Autodesk Fusion 360 part; units mm, degrees
(part 6 of 6)
  line L3972 (32.949444, 239.306805) -> (33.090556, 239.906528)
  line L3973 (28.328056, 253.559028) -> (28.398611, 253.594305)
  line L3974 (29.845, 285.802917) -> (29.809722, 285.697083)
  line L3975 (13.229167, 258.180417) -> (13.193889, 258.497917)
  line L3976 (27.269722, 228.75875) -> (27.199167, 228.864583)
  line L3977 (21.801667, 225.407361) -> (21.872222, 225.477917)
  line L3978 (35.665833, 285.555972) -> (35.736389, 285.59125)
  line L3979 (35.736389, 285.59125) -> (35.771667, 285.661805)
  line L3980 (35.771667, 285.661805) -> (35.806944, 285.873472)
  line L3981 (42.051111, 264.424583) -> (42.156944, 264.283472)
  line L3982 (42.156944, 264.283472) -> (42.2275, 264.248194)
  line L3983 (42.2275, 264.248194) -> (42.298056, 264.248194)
  line L3984 (41.557222, 264.847917) -> (41.733611, 264.812639)
  line L3985 (38.911389, 241.635139) -> (39.017222, 241.599861)
  line L3986 (38.382222, 243.434305) -> (38.311667, 243.68125)
  line L3987 (27.234444, 231.93375) -> (27.340278, 232.004305)
  line L3988 (25.011944, 247.244305) -> (25.611667, 247.385417)
  line L3989 (31.4325, 231.93375) -> (31.467778, 231.863194)
  line L3990 (22.154444, 225.548472) -> (22.754167, 225.548472)
  line L3991 (29.598056, 293.564028) -> (29.598056, 293.422917)
  line L3992 (30.021389, 253.559028) -> (30.056667, 253.594305)
  line L3993 (41.874722, 273.490972) -> (41.345556, 275.325417)
  line L3994 (41.345556, 275.325417) -> (40.781111, 273.490972)
  line L3995 (40.781111, 273.490972) -> (41.874722, 273.490972)
  line L3996 (28.575, 253.559028) -> (28.610278, 253.52375)
  line L3997 (29.809722, 294.763472) -> (27.798889, 294.763472)
  line L3998 (10.830278, 224.63125) -> (10.724444, 224.772361)
  line L3999 (29.421667, 293.21125) -> (29.351111, 293.175972)
  line L4000 (40.287222, 244.034028) -> (40.251944, 243.963472)
  line L4001 (34.6075, 286.367361) -> (34.466389, 286.085139)
  line L4002 (34.466389, 286.085139) -> (34.29, 285.90875)
  line L4003 (27.163889, 289.683472) -> (27.199167, 289.577639)
  line L4004 (31.608889, 225.372083) -> (31.573611, 225.336805)
  line L4005 (24.800278, 289.71875) -> (24.765, 289.648194)
  line L4006 (29.845, 232.004305) -> (31.220833, 232.004305)
  line L4007 (31.220833, 232.004305) -> (31.361944, 231.969028)
  line L4008 (26.246667, 234.826528) -> (25.611667, 234.932361)
  line L4009 (8.643056, 223.149583) -> (8.396111, 223.114305)
  line L4010 (8.396111, 223.114305) -> (6.173611, 223.114305)
  line L4011 (31.467778, 228.899861) -> (31.467778, 228.829305)
  line L4012 (23.530278, 229.852361) -> (23.565556, 229.640694)
  line L4013 (23.212778, 230.169861) -> (23.353889, 230.134583)
  line L4014 (40.3225, 233.239028) -> (40.357778, 233.168472)
  line L4015 (24.024167, 218.034306) -> (25.435278, 218.034306)
  line L4016 (17.674167, 218.034306) -> (19.085278, 218.034306)
  line L4017 (23.600833, 222.549861) -> (19.085278, 218.034306)
  line L4018 (19.085278, 218.034306) -> (24.024167, 218.034306)
  line L4019 (24.024167, 218.034306) -> (28.504444, 222.549861)
  line L4020 (29.351111, 293.175972) -> (29.421667, 293.21125)
  line L4021 (32.208611, 295.292639) -> (32.0675, 295.186805)
  line L4022 (31.785278, 287.249305) -> (31.891111, 286.790694)
  line L4023 (31.891111, 286.790694) -> (32.032222, 286.473194)
  line L4024 (32.032222, 286.473194) -> (32.243889, 286.190972)
  line L4025 (32.596667, 289.542361) -> (32.208611, 289.119028)
  line L4026 (40.181389, 253.20625) -> (40.251944, 253.20625)
  line L4027 (38.311667, 244.245694) -> (38.4175, 244.527917)
  line L4028 (31.220833, 228.723472) -> (29.845, 228.723472)
  line L4029 (23.777222, 289.648194) -> (23.741944, 289.71875)
  line L4030 (41.521944, 263.04875) -> (41.627778, 263.013472)
  line L4031 (30.1625, 294.939861) -> (30.091944, 294.834028)
  line L4032 (27.375556, 250.419305) -> (27.410833, 250.384028)
  line L4033 (27.410833, 250.384028) -> (27.446111, 250.34875)
  line L4034 (28.786667, 234.297361) -> (29.421667, 234.509028)
  line L4035 (29.421667, 234.509028) -> (30.021389, 234.79125)
  line L4036 (38.770278, 243.751805) -> (38.840833, 243.575417)
  line L4037 (35.277778, 273.490972) -> (34.148889, 273.490972)
  line L4038 (37.006389, 261.390694) -> (37.041667, 261.284861)
  line L4039 (29.845, 289.295417) -> (29.845, 285.873472)
  line L4040 (38.205833, 253.170972) -> (38.276389, 253.20625)
  line L4041 (28.151667, 227.17125) -> (28.186944, 227.277083)
  line L4042 (38.488056, 243.257917) -> (38.629167, 243.116805)
  line L4043 (39.087778, 244.915972) -> (38.735, 244.810139)
  line L4044 (38.735, 244.810139) -> (38.4175, 244.527917)
  line L4045 (38.4175, 244.527917) -> (38.311667, 244.245694)
  line L4046 (15.451667, 225.301528) -> (15.522222, 225.336805)
  line L4047 (32.138056, 237.613472) -> (31.75, 237.119583)
  line L4048 (15.522222, 225.336805) -> (15.5575, 225.372083)
  line L4049 (15.5575, 225.372083) -> (15.5575, 225.513194)
  line L4050 (35.771667, 285.661805) -> (35.736389, 285.59125)
  line L4051 (28.151667, 224.807639) -> (28.151667, 227.030139)
  line L4052 (38.205833, 294.834028) -> (38.276389, 294.869305)
  line L4053 (38.276389, 294.869305) -> (38.311667, 294.904583)
  line L4054 (38.311667, 294.904583) -> (38.311667, 295.045694)
  line L4055 (32.279167, 287.390417) -> (32.349722, 287.108194)
  line L4056 (32.349722, 287.108194) -> (32.490833, 286.755417)
  line L4057 (32.138056, 257.898194) -> (31.996944, 257.615972)
  line L4058 (29.633333, 231.93375) -> (29.739167, 232.004305)
  line L4059 (39.6875, 241.705694) -> (39.828611, 241.917361)
  line L4060 (30.656389, 280.722917) -> (30.973889, 280.687639)
  line L4061 (32.032222, 291.235694) -> (32.0675, 291.165139)
  line L4062 (32.0675, 291.165139) -> (32.138056, 291.094583)
  line L4063 (32.138056, 291.094583) -> (32.279167, 291.059305)
  line L4064 (12.170833, 227.312361) -> (12.241389, 227.347639)
  line L4065 (15.5575, 225.513194) -> (15.5575, 225.58375)
  line L4066 (15.5575, 225.58375) -> (15.522222, 225.689583)
  line L4067 (36.477222, 227.030139) -> (36.477222, 227.135972)
  line L4068 (31.079722, 295.292639) -> (30.938611, 295.257361)
  line L4069 (28.222222, 289.754028) -> (28.469167, 289.824583)
  line L4070 (35.489444, 285.59125) -> (35.595278, 285.555972)
  line L4071 (35.348333, 289.507083) -> (35.348333, 285.873472)
  line L4072 (35.348333, 289.648194) -> (35.348333, 289.577639)
  line L4073 (13.899444, 257.157361) -> (13.6525, 257.369028)
  line L4074 (29.245278, 293.705139) -> (27.798889, 293.705139)
  line L4075 (28.151667, 227.030139) -> (28.151667, 227.17125)
  line L4076 (27.093333, 289.365972) -> (27.163889, 289.471805)
  line L4077 (27.163889, 289.471805) -> (27.199167, 289.577639)
  line L4078 (38.911389, 244.386805) -> (38.770278, 244.210417)
  line L4079 (31.855833, 222.549861) -> (34.325278, 222.549861)
  line L4080 (34.325278, 222.549861) -> (34.854444, 222.549861)
  line L4081 (36.300833, 222.549861) -> (37.923611, 222.549861)
  line L4082 (28.539722, 253.594305) -> (28.469167, 253.594305)
  line L4083 (29.280556, 252.112639) -> (28.645556, 253.488472)
  line L4084 (31.4325, 229.040972) -> (31.397222, 229.07625)
  line L4085 (31.397222, 229.07625) -> (31.220833, 229.111528)
  line L4086 (31.220833, 228.723472) -> (31.397222, 228.75875)
  line L4087 (31.573611, 225.336805) -> (31.538333, 225.301528)
  line L4088 (23.741944, 289.365972) -> (23.706667, 289.330694)
  line L4089 (23.706667, 289.330694) -> (23.565556, 289.295417)
  line L4090 (23.565556, 289.295417) -> (23.459722, 289.295417)
  line L4091 (16.121944, 227.100694) -> (16.121944, 227.206528)
  line L4092 (16.121944, 227.206528) -> (16.086667, 227.277083)
  line L4093 (16.086667, 227.277083) -> (16.016111, 227.347639)
  line L4094 (16.016111, 227.347639) -> (15.804444, 227.382917)
  line L4095 (14.393333, 287.637361) -> (14.640278, 287.355139)
  line L4096 (23.001111, 225.477917) -> (23.106944, 225.336805)
  line L4097 (32.208611, 227.206528) -> (32.208611, 227.135972)
  line L4098 (27.516667, 234.085694) -> (28.151667, 234.15625)
  line L4099 (28.151667, 234.15625) -> (28.786667, 234.297361)
  line L4100 (27.410833, 228.723472) -> (27.340278, 228.723472)
  line L4101 (38.840833, 243.010972) -> (38.629167, 243.116805)
  line L4102 (37.076944, 261.567083) -> (37.076944, 261.602361)
  line L4103 (38.170556, 285.59125) -> (38.205833, 285.626528)
  line L4104 (38.205833, 285.626528) -> (38.241111, 285.661805)
  line L4105 (38.241111, 285.661805) -> (38.276389, 285.873472)
  line L4106 (40.181389, 241.564583) -> (39.969722, 241.352917)
  line L4107 (33.690278, 289.789305) -> (33.901944, 289.71875)
  line L4108 (33.901944, 289.71875) -> (34.219444, 289.542361)
  line L4109 (26.211389, 248.232083) -> (25.541111, 248.161528)
  line L4110 (25.541111, 248.161528) -> (24.906111, 247.985139)
  line L4111 (40.075556, 240.788472) -> (40.251944, 240.753194)
  line L4112 (34.995556, 265.377083) -> (34.925, 265.377083)
  line L4113 (38.664444, 241.987917) -> (38.770278, 241.77625)
  line L4114 (41.133889, 264.63625) -> (41.310278, 264.777361)
  line L4115 (39.616944, 242.799305) -> (39.511111, 242.834583)
  line L4116 (38.523333, 253.135694) -> (38.523333, 253.065139)
  line L4117 (28.186944, 227.277083) -> (28.222222, 227.312361)
  line L4118 (30.656389, 256.910417) -> (14.781389, 256.910417)
  line L4119 (31.009167, 289.436528) -> (30.973889, 289.365972)
  line L4120 (26.246667, 253.594305) -> (26.105556, 253.594305)
  line L4121 (26.105556, 253.594305) -> (25.999722, 253.52375)
  line L4122 (6.596944, 281.745972) -> (13.899444, 289.048472)
  line L4123 (22.366111, 245.656805) -> (21.942778, 245.198194)
  line L4124 (21.942778, 245.198194) -> (21.59, 244.669028)
  line L4125 (33.549167, 261.46125) -> (33.513889, 261.355417)
  line L4126 (27.763611, 250.560417) -> (27.728333, 250.595694)
  line L4127 (27.728333, 250.595694) -> (27.693056, 250.66625)
  line L4128 (27.340278, 228.723472) -> (27.269722, 228.75875)
  line L4129 (22.683611, 227.100694) -> (22.930556, 226.889028)
  line L4130 (38.276389, 289.507083) -> (38.276389, 285.873472)
  line L4131 (14.181667, 287.954861) -> (14.393333, 287.637361)
  line L4132 (15.5575, 225.513194) -> (15.5575, 225.372083)
  line L4133 (7.337778, 233.909305) -> (7.443611, 234.262083)
  line L4134 (7.443611, 234.262083) -> (7.584722, 234.579583)
  line L4135 (38.311667, 243.68125) -> (38.276389, 243.928194)
  line L4136 (43.991389, 288.836805) -> (39.698083, 284.522333)
  line L4137 (14.957778, 287.108194) -> (15.310556, 286.967083)
  line L4138 (34.043056, 223.290694) -> (34.113611, 223.220139)
  line L4139 (20.743333, 225.26625) -> (20.778611, 224.94875)
  line L4140 (28.081111, 247.385417) -> (28.716111, 247.244305)
  line L4141 (31.467778, 231.863194) -> (31.467778, 231.827917)
  line L4142 (26.176111, 224.772361) -> (26.176111, 224.63125)
  line L4143 (12.911667, 295.821805) -> (1.446389, 284.391805)
  line L4144 (22.366111, 236.660972) -> (21.942778, 237.119583)
  line L4145 (15.451667, 225.724861) -> (15.522222, 225.689583)
  line L4146 (38.981944, 265.553472) -> (39.0525, 265.624028)
  line L4147 (25.611667, 234.932361) -> (25.011944, 235.073472)
  line L4148 (31.996944, 291.30625) -> (32.032222, 291.235694)
  line L4149 (30.374167, 218.034306) -> (34.854444, 222.549861)
  line L4150 (30.374167, 218.034306) -> (31.785278, 218.034306)
  line L4151 (38.452778, 253.170972) -> (38.523333, 253.135694)
  line L4152 (35.983333, 293.705139) -> (37.429722, 293.705139)
  line L4153 (39.087778, 237.084305) -> (39.0525, 237.154861)
  line L4154 (33.690278, 289.789305) -> (33.408056, 289.824583)
  line L4155 (34.642778, 288.977917) -> (34.6075, 289.08375)
  line L4156 (39.969722, 241.352917) -> (39.6875, 241.211805)
  line L4157 (39.334722, 284.885694) -> (39.698083, 284.522333)
  line L4158 (39.123056, 244.457361) -> (39.37, 244.457361)
  line L4159 (38.911389, 244.386805) -> (39.017222, 244.457361)
  line L4160 (39.017222, 244.457361) -> (39.123056, 244.457361)
  line L4161 (38.735, 243.928194) -> (38.770278, 244.210417)
  line L4162 (24.553333, 286.049861) -> (25.646944, 287.884305)
  line L4163 (31.75, 245.198194) -> (32.138056, 244.669028)
  line L4164 (22.436667, 247.667639) -> (21.872222, 247.244305)
  line L4165 (21.872222, 247.244305) -> (21.343056, 246.785694)
  line L4166 (34.713333, 291.517917) -> (33.760833, 292.823194)
  line L4167 (31.326667, 231.61625) -> (31.397222, 231.651528)
  line L4168 (31.397222, 231.651528) -> (31.467778, 231.722083)
  line L4169 (31.467778, 231.722083) -> (31.467778, 231.827917)
  line L4170 (25.117778, 250.313472) -> (25.153056, 250.313472)
  line L4171 (33.901944, 289.71875) -> (33.690278, 289.789305)
  line L4172 (23.106944, 226.642083) -> (23.106944, 226.53625)
  line L4173 (16.121944, 227.100694) -> (16.086667, 226.994861)
  line L4174 (40.040278, 240.329861) -> (39.511111, 240.329861)
  line L4175 (32.173333, 223.537639) -> (32.0675, 223.643472)
  line L4176 (31.855833, 223.114305) -> (32.102778, 223.149583)
  line L4177 (35.489444, 285.59125) -> (35.418889, 285.626528)
  line L4178 (31.961667, 223.643472) -> (31.891111, 223.643472)
  line L4179 (32.243889, 223.396528) -> (32.208611, 223.467083)
  line L4180 (32.208611, 223.467083) -> (32.173333, 223.537639)
  line L4181 (41.557222, 261.672917) -> (41.768889, 261.708194)
  line L4182 (39.087778, 276.771805) -> (39.193611, 276.736528)
  line L4183 (38.558611, 249.749028) -> (38.558611, 251.93625)
  line L4184 (38.346944, 249.431528) -> (38.4175, 249.466805)
  line L4185 (38.4175, 249.466805) -> (38.488056, 249.502083)
  line L4186 (28.222222, 289.330694) -> (28.433889, 289.295417)
  line L4187 (28.469167, 289.824583) -> (28.222222, 289.754028)
  line L4188 (23.071667, 226.359861) -> (22.965833, 226.289305)
  line L4189 (30.938611, 289.330694) -> (30.691667, 289.295417)
  line L4190 (22.86, 226.254028) -> (22.789444, 226.254028)
  line L4191 (25.964444, 288.44875) -> (25.294167, 289.612917)
  line L4192 (24.835556, 285.59125) -> (24.729722, 285.555972)
  line L4193 (25.752778, 224.984028) -> (25.893889, 225.019305)
  line L4194 (31.996944, 257.615972) -> (31.785278, 257.369028)
  line L4195 (40.251944, 240.753194) -> (40.3225, 240.647361)
  line L4196 (39.405278, 227.100694) -> (39.37, 226.994861)
  line L4197 (29.351111, 251.442361) -> (29.280556, 251.442361)
  line L4198 (37.182778, 261.14375) -> (37.288611, 261.14375)
  line L4199 (37.076944, 261.567083) -> (37.006389, 261.46125)
  line L4200 (37.006389, 261.46125) -> (37.006389, 261.390694)
  line L4201 (34.466389, 223.149583) -> (34.325278, 223.114305)
  line L4202 (6.385278, 223.643472) -> (8.431389, 223.643472)
  line L4203 (8.431389, 223.643472) -> (8.501944, 223.643472)
  line L4204 (32.914167, 227.277083) -> (32.984722, 227.312361)
  line L4205 (14.393333, 287.637361) -> (14.640278, 287.355139)
  line L4206 (14.640278, 287.355139) -> (14.957778, 287.108194)
  line L4207 (23.706667, 285.59125) -> (23.459722, 285.555972)
  line L4208 (23.459722, 285.555972) -> (21.237222, 285.555972)
  line L4209 (21.237222, 285.555972) -> (21.131389, 285.555972)
  line L4210 (41.521944, 263.04875) -> (41.416111, 263.119305)
  line L4211 (30.303611, 253.488472) -> (30.338889, 253.382639)
  line L4212 (23.318611, 246.432917) -> (23.847778, 246.750417)
  line L4213 (37.994167, 295.292639) -> (38.205833, 295.257361)
  line L4214 (16.121944, 227.206528) -> (16.121944, 227.100694)
  line L4215 (26.387778, 223.99625) -> (26.740556, 223.749305)
  line L4216 (5.856111, 227.17125) -> (5.891389, 227.277083)
  line L4217 (5.891389, 227.277083) -> (6.0325, 227.347639)
  line L4218 (31.397222, 228.75875) -> (31.220833, 228.723472)
  line L4219 (18.238611, 225.407361) -> (17.321389, 225.407361)
  line L4220 (18.626667, 225.477917) -> (18.415, 225.442639)
  line L4221 (12.911667, 295.821805) -> (7.972778, 295.821805)
  line L4222 (39.722778, 295.821805) -> (39.334722, 295.821805)
  line L4223 (41.768889, 265.341805) -> (41.980556, 265.27125)
  line L4224 (30.268333, 253.559028) -> (30.303611, 253.488472)
  line L4225 (35.489444, 295.186805) -> (35.630556, 295.292639)
  line L4226 (20.778611, 239.306805) -> (20.6375, 239.906528)
  line L4227 (40.251944, 233.309583) -> (40.3225, 233.239028)
  line L4228 (33.302222, 287.707917) -> (33.3375, 287.849028)
  line L4229 (33.3375, 287.849028) -> (33.372778, 287.919583)
  line L4230 (34.043056, 223.467083) -> (34.043056, 226.85375)
  line L4231 (41.733611, 263.542639) -> (42.2275, 263.542639)
  line L4232 (34.360556, 262.378472) -> (34.925, 264.212917)
  line L4233 (43.991389, 282.486805) -> (43.285833, 281.745972)
  line L4234 (23.459722, 289.824583) -> (23.671389, 289.789305)
  line L4235 (23.671389, 289.789305) -> (23.741944, 289.71875)
  line L4236 (23.741944, 289.71875) -> (23.777222, 289.648194)
  line L4237 (39.37, 250.772083) -> (39.299444, 250.736805)
  line L4238 (29.935, 310.1187) -> (30.643, 310.1187)
  line L4239 (35.088, 310.8259) -> (34.38, 310.8259)
  circle A0 centre (11.541, 282.0025) radius 0.375
  circle A1 centre (31.676, 219.943) radius 0.375
  line L4240 (20.101, 265.429) -> (20.101, 266.137)
  line L4241 (36.176, 278.8525) -> (35.581, 279.4475)
  line L4242 (35.581, 279.4475) -> (34.986, 278.8525)
  circle A2 centre (16.233, 266.73) radius 0.375
  circle A3 centre (26.141, 288.9025) radius 0.375
  circle A4 centre (40.616, 306.9726) radius 0.375
  line L4243 (34.38, 304.4759) -> (34.38, 303.7687)
  line L4244 (26.451, 272.7151) -> (25.743, 272.7151)
  line L4245 (22.541, 277.4415) -> (23.303, 277.4415)
  line L4246 (19.393, 265.429) -> (20.101, 265.429)
  line L4247 (19.393, 260.984) -> (20.101, 260.984)
  line L4248 (25.743, 277.1601) -> (25.743, 276.4529)
  circle A5 centre (33.141, 228.903) radius 0.375
  line L4249 (26.451, 272.0079) -> (26.451, 272.7151)
  circle A6 centre (42.141, 270.6025) radius 0.375
  line L4250 (22.581, 260.627) -> (23.343, 260.627)
  line L4251 (29.935, 304.4759) -> (29.935, 303.7687)
  line L4252 (34.38, 310.8259) -> (34.38, 310.1187)
  circle A7 centre (43.291, 237.353) radius 0.375
  circle A8 centre (17.017, 219.183) radius 0.375
  circle A9 centre (4.391, 272.1525) radius 0.7
  line L4253 (9.191, 262.003) -> (10.591, 260.603)
  line L4254 (19.393, 272.7151) -> (19.393, 272.0079)
  line L4255 (26.451, 266.137) -> (25.743, 266.137)
  line L4256 (3.691, 277.0525) -> (5.091, 275.6525)
  line L4257 (9.191, 266.203) -> (10.591, 264.803)
  line L4258 (26.451, 261.692) -> (25.743, 261.692)
  line L4259 (25.743, 266.137) -> (25.743, 265.429)
  circle A10 centre (9.891, 272.1525) radius 0.7
  line L4260 (35.445, 307.7183) -> (35.445, 306.9563)
  line L4261 (25.743, 276.4529) -> (26.451, 276.4529)
  line L4262 (19.393, 261.692) -> (19.393, 260.984)
  arc A11 (36.093026, 341.539213) -> (-0.103241, 284.387336) centre (143.534, 233.455) ccw
  line L4263 (5.091, 266.203) -> (3.691, 264.803)
  arc A12 (30.216078, 236.039598) -> (23.553913, 236.039603) centre (26.885, 241.145) ccw
  line L4264 (5.091, 272.8525) -> (3.691, 271.4525)
  line L4265 (9.191, 277.0525) -> (10.591, 275.6525)
  line L4266 (34.986, 278.8525) -> (35.581, 278.2575)
  line L4267 (26.451, 260.984) -> (26.451, 261.692)
  circle A13 centre (17.719, 274.883) radius 0.375
  line L4268 (29.935, 303.7687) -> (30.643, 303.7687)
  circle A14 centre (9.791, 289.1525) radius 0.375
  line L4269 (22.541, 266.418) -> (23.303, 266.418)
  line L4270 (20.101, 272.7151) -> (19.393, 272.7151)
  line L4271 (35.064, 307.3373) -> (35.826, 307.3373)
  line L4272 (20.101, 276.4529) -> (20.101, 277.1601)
  line L4273 (20.101, 266.137) -> (19.393, 266.137)
  line L4274 (35.088, 303.7687) -> (35.088, 304.4759)
  line L4275 (19.393, 277.1601) -> (19.393, 276.4529)
  line L4276 (19.393, 266.137) -> (19.393, 265.429)
  line L4277 (35.088, 304.4759) -> (34.38, 304.4759)
  line L4278 (22.962, 261.008) -> (22.962, 260.246)
  line L4279 (19.393, 272.0079) -> (20.101, 272.0079)
  line L4280 (5.091, 262.003) -> (3.691, 260.603)
  circle A15 centre (25.191, 281.4525) radius 0.375
  line L4281 (29.654, 307.6783) -> (29.654, 306.9163)
  line L4282 (9.191, 272.8525) -> (10.591, 271.4525)
  line L4283 (19.393, 276.4529) -> (20.101, 276.4529)
  circle A16 centre (4.391, 265.503) radius 0.7
  line L4284 (3.691, 272.8525) -> (5.091, 271.4525)
  line L4285 (25.743, 261.692) -> (25.743, 260.984)
  line L4286 (26.451, 276.4529) -> (26.451, 277.1601)
  line L4287 (34.38, 310.1187) -> (35.088, 310.1187)
  line L4288 (30.643, 303.7687) -> (30.643, 304.4759)
  circle A17 centre (43.841, 288.9525) radius 0.375
  line L4289 (22.962, 272.0315) -> (22.962, 271.2695)
  line L4290 (26.451, 265.429) -> (26.451, 266.137)
  circle A18 centre (32.991, 249.853) radius 0.375
  line L4291 (45.617, 218.031) -> (45.617, 341.5384)
  line L4292 (34.246, 268.703) -> (34.841, 268.108)
  line L4293 (30.643, 310.1187) -> (30.643, 310.8259)
  circle A19 centre (9.891, 261.303) radius 0.7
  circle A20 centre (9.891, 265.503) radius 0.7
  circle A21 centre (9.364, 219.158) radius 0.375
  circle A22 centre (33.891, 281.4525) radius 0.375
  circle A23 centre (4.391, 261.303) radius 0.7
  circle A24 centre (43.191, 245.753) radius 0.375
  line L4294 (35.581, 278.2575) -> (36.176, 278.8525)
  line L4295 (10.591, 277.0525) -> (9.191, 275.6525)
  line L4296 (25.743, 272.0079) -> (26.451, 272.0079)
  line L4297 (25.441, 300.3525) -> (25.041, 299.9525)
  line L4298 (29.273, 307.2973) -> (30.035, 307.2973)
  line L4299 (25.743, 272.7151) -> (25.743, 272.0079)
  line L4300 (10.591, 266.203) -> (9.191, 264.803)
  line L4301 (34.841, 269.298) -> (34.246, 268.703)
  line L4302 (25.041, 300.3525) -> (25.441, 299.9525)
  line L4303 (25.743, 265.429) -> (26.451, 265.429)
  line L4304 (35.436, 268.703) -> (34.841, 269.298)
  line L4305 (45.617, 341.5384) -> (36.092, 341.5384)
  line L4306 (25.743, 260.984) -> (26.451, 260.984)
  line L4307 (22.922, 266.799) -> (22.922, 266.037)
  circle A25 centre (4.391, 276.3525) radius 0.7
  line L4308 (33.041, 278.2575) -> (33.636, 278.8525)
  circle A26 centre (24.819, 304.2411) radius 0.375
  line L4309 (32.446, 278.8525) -> (33.041, 278.2575)
  line L4310 (22.581, 271.6505) -> (23.343, 271.6505)
  line L4311 (20.101, 261.692) -> (19.393, 261.692)
  line L4312 (3.691, 266.203) -> (5.091, 264.803)
  line L4313 (33.041, 279.4475) -> (32.446, 278.8525)
  circle A27 centre (36.824, 304.1903) radius 0.375
  circle A28 centre (43.641, 281.3525) radius 0.375
  line L4314 (30.643, 310.8259) -> (29.935, 310.8259)
  line L4315 (5.091, 277.0525) -> (3.691, 275.6525)
  circle A29 centre (35.391, 288.9025) radius 0.375
  line L4316 (33.636, 278.8525) -> (33.041, 279.4475)
  circle A30 centre (9.891, 276.3525) radius 0.7
  circle A31 centre (23.912, 219.981) radius 0.375
  line L4317 (34.841, 268.108) -> (35.436, 268.703)
  line L4318 (35.088, 310.1187) -> (35.088, 310.8259)
  line L4319 (-0.103, 284.3884) -> (-0.103, 218.031)
  circle A32 centre (39.616, 219.931) radius 0.375
  line L4320 (-0.103, 218.031) -> (45.617, 218.031)
  line L4321 (30.643, 304.4759) -> (29.935, 304.4759)
  line L4322 (10.591, 262.003) -> (9.191, 260.603)
  line L4323 (22.922, 277.8225) -> (22.922, 277.0605)
  line L4324 (3.691, 262.003) -> (5.091, 260.603)
  line L4325 (20.101, 277.1601) -> (19.393, 277.1601)
  circle A33 centre (18.591, 236.003) radius 0.375
  line L4326 (23.554, 236.04) -> (30.216, 236.04)
  circle A34 centre (42.291, 259.153) radius 0.375
  line L4327 (34.38, 303.7687) -> (35.088, 303.7687)
  line L4328 (20.101, 260.984) -> (20.101, 261.692)
  line L4329 (29.935, 310.8259) -> (29.935, 310.1187)
  line L4330 (10.591, 272.8525) -> (9.191, 271.4525)
  line L4331 (20.101, 272.0079) -> (20.101, 272.7151)
  line L4332 (26.451, 277.1601) -> (25.743, 277.1601)
  circle A35 centre (41.704, 227.215) radius 0.375
  line L4333 (14.781389, 279.722917) -> (30.656389, 279.722917)
  line L4334 (14.193889, 279.135417) -> (14.193889, 258.497917)
  line L4335 (31.243889, 279.135417) -> (31.243889, 258.497917)
  line L4336 (30.656389, 257.910417) -> (14.781389, 257.910417)
  line L4337 (30.656389, 279.722917) -> (31.243889, 279.722917)
  line L4338 (31.243889, 279.135417) -> (31.243889, 279.722917)
  line L4339 (14.781389, 279.722917) -> (14.332148, 279.722917)
  line L4340 (14.332148, 279.722917) -> (14.196325, 279.722917)
  line L4341 (14.196325, 279.722917) -> (14.193889, 279.135417)
  line L4342 (14.781389, 257.910417) -> (14.193889, 257.910417)
  line L4343 (14.193889, 257.910417) -> (14.193889, 258.497917)
  line L4344 (31.243889, 258.497917) -> (31.243889, 257.90808)
  line L4345 (31.243889, 257.90808) -> (30.656389, 257.910417)
  line L4346 (31.243889, 268.816667) -> (14.193889, 268.816667)
  line L4347 (31.312265, 269.316667) -> (14.125513, 269.316667)
  line L4348 (14.125513, 269.316667) -> (14.125513, 268.316667)
  line L4349 (14.125513, 268.316667) -> (31.312265, 268.316667)
  line L4350 (31.312265, 268.316667) -> (31.312265, 269.316667)
  line L4351 (31.312265, 269.316667) -> (14.125513, 268.316667) construction
  line L4352 (14.125513, 269.316667) -> (31.312265, 268.316667) construction
  line L4353 (14.781389, 279.522917) -> (30.656389, 279.522917)
  line L4354 (31.043889, 268.332282) -> (31.043889, 268.316667)
  line L4355 (31.043889, 279.135417) -> (31.043889, 269.516667)
  line L4356 (31.043889, 269.316667) -> (31.043889, 269.301051)
  line L4357 (31.043889, 269.516667) -> (14.393889, 269.516667)
  line L4358 (14.393889, 268.316667) -> (14.393889, 268.332282)
  line L4359 (14.393889, 269.301051) -> (14.393889, 269.316667)
  line L4360 (14.393889, 269.516667) -> (14.393889, 279.135417)
  line L4361 (14.781389, 279.522917) -> (14.393889, 279.522917)
  line L4362 (14.393889, 279.522917) -> (14.393889, 279.135417)
  line L4363 (30.656389, 279.522917) -> (31.043889, 279.522917)
  line L4364 (31.043889, 279.522917) -> (31.043889, 279.135417)
  line L4365 (20.101, 276.4529) -> (25.743, 276.4529)
  line L4366 (25.743, 276.4529) -> (25.743, 272.7151)
  line L4367 (25.743, 272.7151) -> (20.101, 272.7151)
  line L4368 (20.101, 272.7151) -> (20.101, 276.4529)
  line L4369 (14.893889, 279.022917) -> (30.543889, 279.022917)
  line L4370 (30.543889, 279.022917) -> (30.543889, 270.016667)
  line L4371 (30.543889, 269.316667) -> (30.543889, 269.271959)
  line L4372 (30.543889, 268.361374) -> (30.543889, 268.316667)
  line L4373 (14.893889, 268.316667) -> (14.893889, 268.361374)
  line L4374 (14.893889, 269.271959) -> (14.893889, 269.316667)
  line L4375 (14.893889, 270.016667) -> (14.893889, 279.022917)
  line L4376 (30.543889, 270.016667) -> (14.893889, 270.016667)
  circle A36 centre (22.922, 274.584) radius 0.5
  line L4377 (22.718889, 279.022917) -> (22.718889, 274.336667)
  line L4378 (30.543889, 274.519792) -> (22.718889, 274.519792)
  line L4379 (29.968889, 278.519792) -> (15.468889, 278.519792)
  line L4380 (15.468889, 278.519792) -> (15.468889, 270.519792)
  line L4381 (15.468889, 270.519792) -> (29.968889, 270.519792)
  line L4382 (29.968889, 270.519792) -> (29.968889, 278.519792)
  line L4383 (29.968889, 278.519792) -> (15.468889, 270.519792) construction
  line L4384 (15.468889, 278.519792) -> (29.968889, 270.519792) construction
  point P0 (22.718889, 268.816667)
  point P1 (22.718889, 274.519792)
  dimension "d1" = 1
  dimension "d2" = -1
  dimension "d3" = 1
  dimension "d4" = 1
  dimension "d5" = 1
  dimension "d11" = 1.2
  dimension "d24" = 1
  dimension "d25" = 14.5
  dimension "d26" = 8
  constraint parallel L245 L2581
  constraint parallel L1585 L2063
  constraint perpendicular L1276 L4337
  constraint perpendicular L4337 L4338
  constraint parallel L4339 L4340
  constraint perpendicular L4334 L4342
  constraint perpendicular L4336 L4343
  constraint parallel L4335 L4344
  constraint perpendicular L4334 L4346
  constraint horizontal L4347
  constraint perpendicular L4347 L4348
  constraint parallel L4347 L4349
  constraint parallel L4348 L4350
  constraint equal L1585 L3658
  constraint parallel L1276 L4355
  constraint parallel L1585 L4358
  constraint collinear L4354 L4355
  constraint collinear L4355 L4356
  constraint collinear L4358 L4359
  constraint collinear L4359 L4360
  constraint perpendicular L4360 L4361
  constraint perpendicular L4361 L4362
  constraint perpendicular L4355 L4363
  constraint perpendicular L4353 L4364
  constraint horizontal L4365
  constraint vertical L4366
  constraint horizontal L4367
  constraint vertical L4368
  constraint parallel L1585 L4373
  constraint parallel L245 L4369
  constraint parallel L1276 L4370
  constraint collinear L4370 L4371
  constraint collinear L4371 L4372
  constraint collinear L4373 L4374
  constraint collinear L4374 L4375
  constraint perpendicular L4369 L4377
  constraint perpendicular L4377 L4378
  constraint horizontal L4379
  constraint perpendicular L4379 L4380
  constraint parallel L4379 L4381
  constraint parallel L4380 L4382
  measures "d24" diameter of A36
extrude "Extrude1" add sketch "Master Arm Legend Plate" along normal blind 5 contours L167 L245 L306 L332 L418 L654 L1022 L1045 L1256 L1276 L1585 L2061 L2062 L2063 L2064 L2143 L2227 L2411 L2412 L2413 L2414 L2426 L2427 L2428 L2429 L2558 L2567 L2571 L2572 L2573 L2574 L2580 L2581 L2582 L2583 L2820 L2821 L2822 L2823 L3139 L3313 L3314 L3341 L3343 L3345 L3346 L3365 L3381 L3427 L3431 L3438 L3523 L3528 L3535 L3541 L3547 L3582 L3583 L3585 L3586 L3587 L3588 L3658 L3859 L3874 L3970 L3975 L4057 L4060 L4073 L4118 L4194 | L4334 L4335 L4346 L4347 | L4334 L4335 L4346 L4349 picked at (25.364722, 257.24375) picked at (20.110556, 268.983333) picked at (20.110556, 268.65) makes body 1
ref_plane "WorkPlane1" through (-2.281111, -6.183333, 2) normal (0, 0, 1) x (1, 0, 0)
sketch "Sketch3" plane through (-2.281111, -6.183333, 2) normal (0, 0, 1) x (1, 0, 0)
  line L0 (8.767455, -11.15191) -> (-8.767455, -11.15191)
  line L1 (-8.767455, -11.15191) -> (-8.767455, 11.15191)
  line L2 (-8.767455, 11.15191) -> (8.767455, 11.15191)
  line L3 (8.767455, 11.15191) -> (8.767455, -11.15191)
  line L4 (8.767455, -11.15191) -> (-8.767455, 11.15191) construction
  line L5 (-8.767455, -11.15191) -> (8.767455, 11.15191) construction
  line L6 (10.601651, -12.65595) -> (-10.601651, -12.65595)
  line L7 (-10.601651, -12.65595) -> (-10.601651, 12.65595)
  line L8 (-10.601651, 12.65595) -> (10.601651, 12.65595)
  line L9 (10.601651, 12.65595) -> (10.601651, -12.65595)
  line L10 (10.601651, -12.65595) -> (-10.601651, 12.65595) construction
  line L11 (-10.601651, -12.65595) -> (10.601651, 12.65595) construction
  constraint horizontal L0
  constraint perpendicular L0 L1
  constraint parallel L0 L2
  constraint parallel L1 L3
  constraint coincident L4 origin
  constraint coincident L5 origin
  constraint horizontal L6
  constraint perpendicular L6 L7
  constraint parallel L6 L8
  constraint parallel L7 L9
  constraint coincident L10 origin
  constraint coincident L11 origin
extrude "Extrude2" add sketch "Sketch3" against normal blind 2 contours L6 L7 L8 L9 picked at (-9.990252, -3.717303) bodies 1
extrude "Extrude3" add sketch "Master Arm Legend Plate" along normal blind 6 separate body contours L4353 L4355 L4357 L4360 L4361 L4362 L4363 L4364 picked at (22.718889, 279.35625) makes body 2
extrude "Extrude4" add sketch "Master Arm Legend Plate" along normal blind 1 contours L4244 L4249 L4296 L4299 | L4254 L4270 L4279 L4331 | L4272 L4275 L4283 L4325 | L4365 L4366 L4367 L4368 L4377 L4378 L4379 L4380 L4381 L4382 | L4365 L4366 L4367 L4368 A36 L4377 L4378 | L4365 L4366 A36 L4377 L4378 | L4248 L4261 L4286 L4332 | L4365 L4366 L4377 L4378 L4379 L4382 | L4369 L4370 L4377 L4378 L4379 L4382 | L4369 L4370 L4375 L4376 L4377 L4378 L4379 L4380 L4381 L4382 | A36 L4377 L4378 | A36 L4377 L4378 | A13 picked at (25.979, 272.479367) picked at (19.865, 272.243633) picked at (19.865, 276.688633) picked at (28.796259, 272.584894) picked at (20.874785, 274.577734) picked at (24.954421, 275.254472) picked at (25.979, 276.924367) picked at (28.796259, 276.497494) picked at (30.352222, 277.354167) picked at (15.085556, 275.853125) picked at (23.166034, 274.67823) picked at (23.179872, 274.49553) picked at (17.61572, 274.953415) bodies 2
extrude "Extrude5" add sketch "Master Arm Legend Plate" along normal blind 3 contours L4369 L4370 L4377 L4378 L4379 L4382 | L4369 L4370 L4375 L4376 L4377 L4378 L4379 L4380 L4381 L4382 picked at (30.352222, 277.354167) picked at (15.085556, 275.853125) bodies 2
sketch "Sketch1" plane through (0, 0, 0) normal (0, 1, 0) x (1, 0, 0) in component "PUSH BUTTON SUPPORT v4"
  line L0 (2.815, 2.25) -> (-2.815, 2.25)
  line L1 (-2.815, 2.25) -> (-2.815, -2.25)
  line L2 (-2.815, -2.25) -> (2.815, -2.25)
  line L3 (2.815, -2.25) -> (2.815, 2.25)
  line L4 (2.815, 2.25) -> (-2.815, -2.25) construction
  line L5 (-2.815, 2.25) -> (2.815, -2.25) construction
  line L6 (3.815, 3.25) -> (-3.815, 3.25)
  line L7 (-3.815, 3.25) -> (-3.815, -3.25)
  line L8 (-3.815, -3.25) -> (3.815, -3.25)
  line L9 (3.815, -3.25) -> (3.815, 3.25)
  line L10 (3.815, 3.25) -> (-3.815, -3.25) construction
  line L11 (-3.815, 3.25) -> (3.815, -3.25) construction
  line L12 (1, 1.85) -> (-1, 1.85)
  line L13 (1, 1.85) -> (-1, -1.85) construction
  line L14 (-1, 1.85) -> (1, -1.85) construction
  line L15 (-0.994265, -2.25) -> (1, -2.25)
  line L16 (1, -2.25) -> (1, -1.85)
  line L17 (1, -1.85) -> (-0.994265, -1.85)
  line L18 (-0.994265, -1.85) -> (-0.994265, -2.25)
  line L19 (1, 1.85) -> (1, 2.25)
  line L20 (1, 2.25) -> (-1, 2.25)
  line L21 (-1, 2.25) -> (-1, 1.85)
  line L22 (-2.815, -2.25) -> (-2.515, -2.25)
  line L23 (-2.515, -2.25) -> (-2.515, 2.25)
  line L24 (-2.515, 2.25) -> (-2.815, 2.25)
  line L25 (-2.815, 2.25) -> (-2.815, -2.25)
  line L26 (2.815, -2.25) -> (2.515, -2.25)
  line L27 (2.515, -2.25) -> (2.515, 2.25)
  line L28 (2.515, 2.25) -> (2.815, 2.25)
  line L29 (2.815, 2.25) -> (2.815, -2.25)
  dimension "d1_1" = 5.63
  dimension "d2_1" = 4.5
  dimension "d3_1" = 7.63
  dimension "d4_1" = 6.5
  dimension "d7_1" = 2
  dimension "d8_1" = 3.7
  dimension "d11_1" = 0.3
  dimension "d12" = 0.3
  constraint horizontal L0
  constraint perpendicular L0 L1
  constraint parallel L0 L2
  constraint parallel L1 L3
  constraint coincident L4 origin
  constraint coincident L5 origin
  constraint horizontal L6
  constraint perpendicular L6 L7
  constraint parallel L6 L8
  constraint parallel L7 L9
  constraint coincident L10 origin
  constraint coincident L11 origin
  constraint horizontal L12
  constraint coincident L13 origin
  constraint coincident L14 origin
  constraint horizontal L15
  constraint vertical L16
  constraint horizontal L17
  constraint vertical L18
  constraint vertical L19
  constraint horizontal L20
  constraint vertical L21
  constraint coincident L0 L19.end
  constraint horizontal L22
  constraint vertical L23
  constraint horizontal L24
  constraint vertical L25
  constraint horizontal L26
  constraint vertical L27
  constraint horizontal L28
  constraint vertical L29
  measures "d1_1" distance of L1.end L2.end
  measures "d2_1" distance of L0.end L1.end
  measures "d3_1" distance of L7.end L8.end
  measures "d4_1" distance of L6.end L7.end
  measures "d7_1" distance of L13.end L14.end
  measures "d8_1" distance of L12.end L13.end
  measures "d11_1" distance of L1.end L22.end
  measures "d12" distance of L2.end L26.end
extrude "Extrude1'" add sketch "Sketch1" along normal blind 5 separate body contours L6 L7 L8 L9 picked at (-0.331422, -2.916667) makes body 3 in component "PUSH BUTTON SUPPORT v4"
extrude "Extrude2'" add sketch "Sketch1" along normal blind 5 contours L0 L12 L19 L20 L21 | L2 L15 L16 L17 L18 picked at (-0.333333, 2.116667) picked at (0.335245, -2.116667) bodies 3 in component "PUSH BUTTON SUPPORT v4"
extrude "Extrude3'" add sketch "Sketch1" along normal blind 1.8 contours L0 L2 L3 L26 L27 L28 L29 | L0 L1 L2 L22 L23 L24 L25 picked at (2.615, 0.75) picked at (-2.715, 0.75) bodies 3 in component "PUSH BUTTON SUPPORT v4"
chamfer "Chamfer1" distance 0.3 angle 45 2 edges at (-2.515, 1.8, 0) (2.515, 1.8, 0) on bodies 3 in component "PUSH BUTTON SUPPORT v4"
chamfer "Chamfer3" distance 0.9 distance2 0.3 1 edges at (-2.515, 0, 0) measured on face at (-2.515, 0.50002, 0.75) on bodies 3 in component "PUSH BUTTON SUPPORT v4"
chamfer "Chamfer4" distance 0.3 distance2 1 1 edges at (2.515, 0, 0) measured on face at (3.381667, 0, 0.75) on bodies 3 in component "PUSH BUTTON SUPPORT v4"
sketch "Sketch2" plane through (0, 0, 3.25) normal (0, 0, 1) x (-1, 0, 0) in component "PUSH BUTTON SUPPORT v4"
  line L0 (3.815, 0) -> (-3.815, 0)
  line L1 (-3.815, 0) -> (-3.815, -5)
  line L2 (-3.815, -5) -> (3.815, -5)
  line L3 (3.815, -5) -> (3.815, 0)
  line L4 (-2.81825, -1.967525) -> (2.836671, -1.967525)
  line L5 (2.836671, -1.967525) -> (2.836671, -2.718821)
  line L6 (2.836671, -2.718821) -> (-2.81825, -2.718821)
  line L7 (-2.81825, -2.718821) -> (-2.81825, -1.967525)
  constraint horizontal L4
  constraint vertical L5
  constraint horizontal L6
  constraint vertical L7
extrude "Extrude4'" add sketch "Sketch2" against normal blind 6.5 contours L4 L5 L6 L7 picked at (-0.933276, -2.217957) bodies 3 in component "PUSH BUTTON SUPPORT v4"
chamfer "Chamfer2" [suppressed] in component "PUSH BUTTON SUPPORT v4"
copy_body "CutPasteBodies1" bodies 2 removing the originals makes body 4 in component "Component"
combine "Combine1" operation add target body 3 tool bodies 4 body 4 seen with x (1, 0, 0) y (0, 0, -1) z (0, 1, 0) at (2.07, 3.986184, -0.383757) in component "PUSH BUTTON SUPPORT v4"
delete_face "DeleteFace1" 1 faces at (-1.271667, 1.328728, 3.25) on bodies 3 in component "PUSH BUTTON SUPPORT v4"
sketch "Sketch1 (2)" plane through (0, 0, 0) normal (0, 1, 0) x (1, 0, 0) in component "PUSH BUTTON SUPPORT v7"
  line L0 (2.815, 2.25) -> (-2.815, 2.25)
  line L1 (-2.815, 2.25) -> (-2.815, -2.25)
  line L2 (-2.815, -2.25) -> (2.815, -2.25)
  line L3 (2.815, -2.25) -> (2.815, 2.25)
  line L4 (2.815, 2.25) -> (-2.815, -2.25) construction
  line L5 (-2.815, 2.25) -> (2.815, -2.25) construction
  line L6 (3.815, 3.25) -> (-3.815, 3.25)
  line L7 (-3.815, 3.25) -> (-3.815, -3.25)
  line L8 (-3.815, -3.25) -> (3.815, -3.25)
  line L9 (3.815, -3.25) -> (3.815, 3.25)
  line L10 (3.815, 3.25) -> (-3.815, -3.25) construction
  line L11 (-3.815, 3.25) -> (3.815, -3.25) construction
  line L12 (1, 1.85) -> (-1, 1.85)
  line L13 (1, 1.85) -> (-1, -1.85) construction
  line L14 (-1, 1.85) -> (1, -1.85) construction
  line L15 (-0.994265, -2.25) -> (1, -2.25)
  line L16 (1, -2.25) -> (1, -1.85)
  line L17 (1, -1.85) -> (-0.994265, -1.85)
  line L18 (-0.994265, -1.85) -> (-0.994265, -2.25)
  line L19 (1, 1.85) -> (1, 2.25)
  line L20 (1, 2.25) -> (-1, 2.25)
  line L21 (-1, 2.25) -> (-1, 1.85)
  line L22 (-2.815, -2.25) -> (-2.515, -2.25)
  line L23 (-2.515, -2.25) -> (-2.515, 2.25)
  line L24 (-2.515, 2.25) -> (-2.815, 2.25)
  line L25 (-2.815, 2.25) -> (-2.815, -2.25)
  line L26 (2.815, -2.25) -> (2.515, -2.25)
  line L27 (2.515, -2.25) -> (2.515, 2.25)
  line L28 (2.515, 2.25) -> (2.815, 2.25)
  line L29 (2.815, 2.25) -> (2.815, -2.25)
  dimension "d1_2" = 5.63
  dimension "d2_2" = 4.5
  dimension "d3_2" = 7.63
  dimension "d4_2" = 6.5
  dimension "d7_2" = 2
  dimension "d8_2" = 3.7
  dimension "d11_2" = 0.3
  dimension "d12_1" = 0.3
  constraint horizontal L0
  constraint perpendicular L0 L1
  constraint parallel L0 L2
  constraint parallel L1 L3
  constraint coincident L4 origin
  constraint coincident L5 origin
  constraint horizontal L6
  constraint perpendicular L6 L7
  constraint parallel L6 L8
  constraint parallel L7 L9
  constraint coincident L10 origin
  constraint coincident L11 origin
  constraint horizontal L12
  constraint coincident L13 origin
  constraint coincident L14 origin
  constraint horizontal L15
  constraint vertical L16
  constraint horizontal L17
  constraint vertical L18
  constraint vertical L19
  constraint horizontal L20
  constraint vertical L21
  constraint coincident L0 L19.end
  constraint horizontal L22
  constraint vertical L23
  constraint horizontal L24
  constraint vertical L25
  constraint horizontal L26
  constraint vertical L27
  constraint horizontal L28
  constraint vertical L29
  measures "d1_2" distance of L1.end L2.end
  measures "d2_2" distance of L0.end L1.end
  measures "d3_2" distance of L7.end L8.end
  measures "d4_2" distance of L6.end L7.end
  measures "d7_2" distance of L13.end L14.end
  measures "d8_2" distance of L12.end L13.end
  measures "d11_2" distance of L1.end L22.end
  measures "d12_1" distance of L2.end L26.end
extrude "Extrude1''" add sketch "Sketch1 (2)" along normal blind 5 separate body contours L6 L7 L8 L9 picked at (-0.331422, -2.916667) makes body 5 in component "PUSH BUTTON SUPPORT v7"
extrude "Extrude2''" add sketch "Sketch1 (2)" along normal blind 5 contours L0 L12 L19 L20 L21 | L2 L15 L16 L17 L18 picked at (-0.333333, 2.116667) picked at (0.335245, -2.116667) bodies 5 in component "PUSH BUTTON SUPPORT v7"
extrude "Extrude3''" add sketch "Sketch1 (2)" along normal blind 1.8 contours L0 L2 L3 L26 L27 L28 L29 | L0 L1 L2 L22 L23 L24 L25 picked at (2.615, 0.75) picked at (-2.715, 0.75) bodies 5 in component "PUSH BUTTON SUPPORT v7"
chamfer "Chamfer1'" distance 0.3 angle 45 2 edges at (-2.515, 1.8, 0) (2.515, 1.8, 0) on bodies 5 in component "PUSH BUTTON SUPPORT v7"
chamfer "Chamfer3'" distance 0.9 distance2 0.3 1 edges at (-2.515, 0, 0) measured on face at (-2.515, 0.50002, 0.75) on bodies 5 in component "PUSH BUTTON SUPPORT v7"
chamfer "Chamfer4'" distance 0.3 distance2 1 1 edges at (2.515, 0, 0) measured on face at (3.381667, 0, 0.75) on bodies 5 in component "PUSH BUTTON SUPPORT v7"
sketch "Sketch2 (2)" plane through (0, 0, 3.25) normal (0, 0, 1) x (-1, 0, 0) in component "PUSH BUTTON SUPPORT v7"
  line L0 (3.815, 0) -> (-3.815, 0)
  line L1 (-3.815, 0) -> (-3.815, -5)
  line L2 (-3.815, -5) -> (3.815, -5)
  line L3 (3.815, -5) -> (3.815, 0)
  line L4 (-2.81825, -1.967525) -> (2.836671, -1.967525)
  line L5 (2.836671, -1.967525) -> (2.836671, -2.718821)
  line L6 (2.836671, -2.718821) -> (-2.81825, -2.718821)
  line L7 (-2.81825, -2.718821) -> (-2.81825, -1.967525)
  constraint horizontal L4
  constraint vertical L5
  constraint horizontal L6
  constraint vertical L7
extrude "Extrude4''" add sketch "Sketch2 (2)" against normal blind 6.5 contours L4 L5 L6 L7 picked at (-0.933276, -2.217957) bodies 5 in component "PUSH BUTTON SUPPORT v7"
sketch "Sketch3 (2)" plane through (0, 1.967525, 0) normal (0, -1, 0) x (1, 0, 0) in component "PUSH BUTTON SUPPORT v7"
  line L0 (-1, -1.85) -> (1, -1.85)
  line L1 (1, -1.85) -> (1, -2.25)
  line L2 (1, -2.25) -> (2.815, -2.25)
  line L3 (2.815, -2.25) -> (2.815, 2.25)
  line L4 (2.815, 2.25) -> (1, 2.25)
  line L5 (1, 2.25) -> (1, 1.85)
  line L6 (1, 1.85) -> (-0.994265, 1.85)
  line L7 (-0.994265, 1.85) -> (-0.994265, 2.25)
  line L8 (-0.994265, 2.25) -> (-2.815, 2.25)
  line L9 (-2.815, 2.25) -> (-2.815, -2.25)
  line L10 (-2.815, -2.25) -> (-1, -2.25)
  line L11 (-1, -2.25) -> (-1, -1.85)
  circle A0 centre (0, 0) radius 1.019835
  constraint coincident A0.centre origin
extrude "Extrude5'" cut sketch "Sketch3 (2)" against normal blind 6.5 contours A0 picked at (-0.371624, 0.422719) bodies 5 in component "PUSH BUTTON SUPPORT v7"
extrude "Extrude6" cut 1 faces at (-0.331422, 5, 2.916667) along direction (0, -1, 0) blind 2 on bodies 5 bodies 5 in component "PUSH BUTTON SUPPORT v7"
extrude "Extrude7" cut 1 faces at (1, 0.655842, -1.983333) along direction (-1, 0, 0) blind 0.3 on bodies 5 bodies 5 in component "PUSH BUTTON SUPPORT v7"
extrude "Extrude8" cut 1 faces at (1, 0.655842, 2.116667) along direction (-1, 0, 0) blind 0.3 on bodies 5 bodies 5 in component "PUSH BUTTON SUPPORT v7"
extrude "Extrude9" cut 1 faces at (-1, 0.655842, -2.116667) along direction (1, 0, 0) blind 0.3 on bodies 5 bodies 5 in component "PUSH BUTTON SUPPORT v7"
extrude "Extrude10" cut 1 faces at (-0.994265, 0.655842, 1.983333) along direction (1, 0, 0) blind 0.3 on bodies 5 bodies 5 in component "PUSH BUTTON SUPPORT v7"
extrude "Extrude11" cut 2 faces at (-1.305, 0.955842, -2.25) (1.305, 0.989175, -2.25) along direction (0, 0, -1) blind 0.3 on bodies 5 bodies 5 in component "PUSH BUTTON SUPPORT v7"
extrude "Extrude12" cut 2 faces at (-1.301176, 0.955842, 2.25) (1.305, 0.989175, 2.25) along direction (0, 0, 1) blind 0.3 on bodies 5 bodies 5 in component "PUSH BUTTON SUPPORT v7"
extrude "Extrude13" cut 1 faces at (-3.481667, 0, -0.85) along direction (0, 1, 0) blind 0.5 on bodies 5 bodies 5 in component "PUSH BUTTON SUPPORT v7"
extrude "Extrude14" cut 1 faces at (-2.815, 0.166667, -0.85) along direction (1, 0, 0) blind 8 on bodies 5 bodies 5 in component "PUSH BUTTON SUPPORT v7"
extrude "Extrude15" cut 2 faces at (2.81498, 1.8, 0.85) (2.71496, 1.70002, -0.85) along direction (0.70710678, -0.70710678, 0) blind 0.3 on bodies 5 bodies 5 in component "PUSH BUTTON SUPPORT v7"
extrude "Extrude16" cut 2 faces at (-2.81498, 1.8, -0.85) (-2.71496, 1.70002, -0.85) along direction (-0.70710678, -0.70710678, 0) blind 0.3 on bodies 5 bodies 5 in component "PUSH BUTTON SUPPORT v7"
extrude "Extrude17" cut 1 faces at (2.565, 0.833333, 0.85) along direction (0.95782629, 0.28734789, 0) blind 0.1 on bodies 5 bodies 5 in component "PUSH BUTTON SUPPORT v7"
extrude "Extrude18" cut 1 faces at (-2.559444, 0.766667, 0.85) along direction (-0.9486833, 0.31622777, 0) blind 0.1 on bodies 5 bodies 5 in component "PUSH BUTTON SUPPORT v7"
extrude "Extrude19" cut 1 faces at (2.515, 1.166687, 0.85) along direction (1, 0, 0) blind 0.1 on bodies 5 bodies 5 in component "PUSH BUTTON SUPPORT v7"
extrude "Extrude20" cut 1 faces at (-2.515, 1.10002, 0.85) along direction (-1, 0, 0) blind 0.1 on bodies 5 bodies 5 in component "PUSH BUTTON SUPPORT v7"
extrude "Extrude21" cut 1 faces at (-2.815, 1.911683, -0.85) along direction (-1, 0, 0) blind 0.2 on bodies 5 bodies 5 in component "PUSH BUTTON SUPPORT v7"
extrude "Extrude22" cut 1 faces at (2.815, 1.911683, -0.85) along direction (1, 0, 0) blind 0.2 on bodies 5 bodies 5 in component "PUSH BUTTON SUPPORT v7"
extrude "Extrude23" cut 1 faces at (-0.7, 0.989175, -2.316667) along direction (1, 0, 0) blind 0.5 on bodies 5 bodies 5 in component "PUSH BUTTON SUPPORT v7"
extrude "Extrude24" cut 1 faces at (-0.694265, 1.47835, 2.316667) along direction (1, 0, 0) blind 0.5 on bodies 5 bodies 5 in component "PUSH BUTTON SUPPORT v7"
extrude "Extrude25" cut 1 faces at (0.7, 0.989175, 2.316667) along direction (-1, 0, 0) blind 0.5 on bodies 5 bodies 5 in component "PUSH BUTTON SUPPORT v7"
extrude "Extrude26" cut 1 faces at (0.7, 1.47835, -2.316667) along direction (-1, 0, 0) blind 0.5 on bodies 5 bodies 5 in component "PUSH BUTTON SUPPORT v7"
extrude "Extrude27" cut 1 faces at (0.068578, 0.989175, 1.85) along direction (0, 0, 1) blind 0.2 on bodies 5 bodies 5 in component "PUSH BUTTON SUPPORT v7"
extrude "Extrude28" cut 1 faces at (0.066667, 0.989175, -1.85) along direction (0, 0, -1) blind 0.2 on bodies 5 bodies 5 in component "PUSH BUTTON SUPPORT v7"
extrude "Extrude29" cut 2 faces at (1.005, 1.289195, -2.55) (-1.005, 1.289195, -2.55) along direction (0, 0, -1) blind 0.1 on bodies 5 bodies 5 in component "PUSH BUTTON SUPPORT v7"
extrude "Extrude30" cut 2 faces at (-1.001176, 1.289195, 2.55) (1.005, 1.289195, 2.55) along direction (0, 0, 1) blind 0.1 on bodies 5 bodies 5 in component "PUSH BUTTON SUPPORT v7"
chamfer "Chamfer2'" [suppressed] in component "PUSH BUTTON SUPPORT v7"
move_body "Move1" bodies 3 to x (1, 0, 0) y (0, 1, 0) z (0, 0, 1) at (2, 0, 0) in component "PUSH BUTTON SUPPORT v4"
fillet "Fillet1" radius 1 4 edges at (-6.536111, 6.986184, 5.099576) (10.113889, 6.986184, 5.099576) (10.113889, 6.986184, -4.906674) (-6.536111, 6.986184, -4.906674) on bodies 3 in component "PUSH BUTTON SUPPORT v4"
extrude "Extrude5''" add 1 faces at (4.397222, 8.986184, 4.599576) along direction (0, 0, -1) blind 0.3 on bodies 3 bodies 3 in component "PUSH BUTTON SUPPORT v4"
extrude "Extrude6'" add 1 faces at (9.613889, 8.986184, 1.397493) along direction (-1, 0, 0) blind 0.3 on bodies 3 bodies 3 in component "PUSH BUTTON SUPPORT v4"
extrude "Extrude7'" add 1 faces at (-0.919444, 7.986184, -4.406674) along direction (0, 0, 1) blind 0.3 on bodies 3 bodies 3 in component "PUSH BUTTON SUPPORT v4"
extrude "Extrude8'" add 1 faces at (-6.036111, 7.986184, 1.497493) along direction (1, 0, 0) blind 0.3 on bodies 3 bodies 3 in component "PUSH BUTTON SUPPORT v4"
extrude "Extrude9'" add 1 faces at (4.205556, 5.652851, -3.903549) along direction (0, 0, 1) blind 0.3 on bodies 3 bodies 3 in component "PUSH BUTTON SUPPORT v4"
extrude "Extrude10'" add 1 faces at (-5.461111, 5.652851, -1.036882) along direction (1, 0, 0) blind 0.3 on bodies 3 bodies 3 in component "PUSH BUTTON SUPPORT v4"
extrude "Extrude11'" add 1 faces at (4.305556, 6.319518, 4.096451) along direction (0, 0, -1) blind 0.3 on bodies 3 bodies 3 in component "PUSH BUTTON SUPPORT v4"
extrude "Extrude12'" add 1 faces at (9.038889, 5.652851, 1.329785) along direction (-1, 0, 0) blind 0.3 on bodies 3 bodies 3 in component "PUSH BUTTON SUPPORT v4"
extrude "Extrude7''" [suppressed]
extrude "Extrude6''" [suppressed]
component "PUSH BUTTON SUPPORT v4" placed x (1, 0, 0) y (0, 0, 1) z (0, -1, 0) at (-2.07, -0.383757, -3.986184)
component "Component" placed x (1, 0, 0) y (0, 1, 0) z (0, 0, 1) at (0, 0, 0)
component "PUSH BUTTON SUPPORT v7" placed x (1, 0, 0) y (0, 0, 1) z (0, -1, 0) at (-0.25, -0.5, -2.5)
hidden bodies 1
named bodies: "Outter Shell", "A/A Button"
